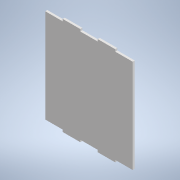
# Autodesk Inventor part: achterbak
Saved by Autodesk Inventor 2021 (Build 250183000, 183)
## iProperties
Created: 2022-02-02
Part Number: achterbak
Material: Generic
Document SubType Name: Modeling
Designer: ryan
Density: 1 g/cm^3
Appearance: Default
Author: ryan
Autodesk Inventor part; units mm, degrees
ref_plane "YZ Plane" through (0, 0, 0) normal (1, 0, 0) x (0, 1, 0)
ref_plane "XZ Plane" through (0, 0, 0) normal (0, 1, 0) x (-1, 0, 0)
ref_plane "XY Plane" through (0, 0, 0) normal (0, 0, 1) x (1, 0, 0)
sketch "Sketch1" plane through (0, 0, 0) normal (0, 0, 1) x (1, 0, 0)
  line L0 (0, 0) -> (0, -3)
  line L1 (0, -3) -> (25, -3)
  line L2 (0, -3) -> (25, -3) construction
  line L3 (25, -3) -> (-100, -3)
  line L4 (-100, -3) -> (-100, 67)
  line L5 (-100, 67) -> (25, 67)
  line L6 (25, 67) -> (25, -3)
  line L7 (0, 0) -> (-25, 0)
  line L8 (-25, 0) -> (-25, -3)
  line L9 (-25, -3) -> (0, -3)
  line L10 (0, -3) -> (0, 0)
  line L11 (-25, 0) -> (-50, 0)
  line L12 (-50, 0) -> (-50, -3)
  line L13 (-50, -3) -> (-25, -3)
  line L14 (-25, -3) -> (-25, 0)
  line L15 (-50, 0) -> (-75, 0)
  line L16 (-75, 0) -> (-75, -3)
  line L17 (-75, -3) -> (-50, -3)
  line L18 (-50, -3) -> (-50, 0)
  line L19 (25, 0) -> (-100, 0)
  line L20 (-75, 0) -> (-100, 0)
  dimension "d0" = 3
  dimension "d1" = 25
  dimension "d2" = 0
  dimension "d3" = 125
  dimension "d4" = 70
  dimension "d5" = 25
  dimension "d6" = 3
  dimension "d7" = 25
  dimension "d8" = 3
  dimension "d9" = 25
  dimension "d10" = 3
  constraints: 42 end point, 8 parallel, 6 horizontal, 6 perpendicular, 2 point on line, 1 collinear, 1 vertical
  measures "d0" distance of L0.start L0.end
  measures "d1" distance of L0.end L1.end
  measures "d2" distance between parallel lines of L1 L2
  measures "d3" distance of L4.end L5.end
  measures "d4" distance of L3.end L4.end
  measures "d5" distance of L9.end L8.end
  measures "d6" distance of L8.end L7.end
  measures "d7" distance of L13.end L12.end
  measures "d8" distance of L12.end L11.end
  measures "d9" distance of L17.end L16.end
  measures "d10" distance of L16.end L15.end
extrude "Extrusion1" add sketch "Sketch1" along normal blind 3 contours L0 L3 L8 L7 | L7 L11 L15 L19 L4 L5 L6 | L12 L3 L16 L15
mirror "Mirror1" about plane through (25, 67, 0) normal (0, 1, 0) of "Extrusion1"
body "Solid1"
